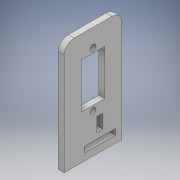
# Autodesk Inventor part: muñeca5
Saved by Autodesk Inventor 2018 (Build 220112000, 112)
## iProperties
Created: 2020-03-11
Part Number: muñeca5
Material: Genérico
Document SubType Name: Modeling
Designer: david
Density: 1 g/cm^3
Appearance: Valor por defecto
Author: david
Autodesk Inventor part; units mm, degrees
ref_plane "YZ Plane" through (0, 0, 0) normal (1, 0, 0) x (0, 1, 0)
ref_plane "XZ Plane" through (0, 0, 0) normal (0, 1, 0) x (-1, 0, 0)
ref_plane "XY Plane" through (0, 0, 0) normal (0, 0, 1) x (1, 0, 0)
sketch "Boceto1" plane through (0, 0, 0) normal (1, 0, 0) x (0, 1, 0)
  line L0 (8, 0) -> (8, -3)
  line L1 (8, -3) -> (-8, -3)
  line L2 (-8, -3) -> (-8, 0)
  line L3 (8, 0) -> (-8, 0)
  line L4 (-18.175, -6.5) -> (11.175, -6.5)
  line L5 (1.5, 3) -> (1.5, 10)
  line L6 (1.5, 10) -> (-1.5, 10)
  line L7 (-1.5, 10) -> (-1.5, 3)
  line L8 (-1.5, 3) -> (1.5, 3)
  line L9 (-9.5, 39) -> (2.5, 39)
  line L10 (2.5, 39) -> (2.5, 16)
  line L11 (-9.5, 39) -> (-9.5, 16)
  line L12 (-9.5, 16) -> (2.5, 16)
  circle A0 centre (-3.5, 41.5) radius 1.5
  circle A1 centre (-3.5, 13.5) radius 1.5
  line L13 (11.175, -6.5) -> (11.175, 45.5)
  line L14 (-18.175, 45.5) -> (-18.175, -6.5)
  line L15 (2.5, 23.4783) -> (2.5, 27.5)
  line L16 (6.175, 50.5) -> (1.5, 50.5)
  line L17 (-8.5, 50.5) -> (-13.175, 50.5)
  line L18 (1.5, 50.5) -> (-8.5, 50.5)
  arc A2 (-13.175, 50.5) -> (-18.175, 45.5) centre (-13.175, 45.5) ccw
  arc A3 (11.175, 45.5) -> (6.175, 50.5) centre (6.175, 45.5) ccw
  point P0 (11.175, 50.5)
  point P1 (-18.175, 50.5)
  dimension "d28" = 5
  constraints: 38 end point, 11 perpendicular, 4 centre point, 4 point on circle, 4 point on line, 4 tangent, 3 vertical, 2 horizontal, 1 equal radius
  measures "d28" radius of A2
extrude "Extrusión1" add sketch "Boceto1" along normal blind 3
